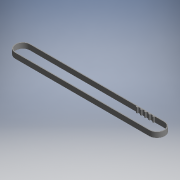
# Autodesk Inventor part: TBN154XL025_info-1-11-11
Saved by Autodesk Inventor 2017.3 (Build 213256000, 256)
## iProperties
Part Number: TBN154XL025_info-1-11-11
Material: Generic
Catalog Web Link: www.cadenas.de
Description: TBN__XL, TUN__XL-Timing Belts XL (Pitch : 5.08mm)
Vendor: MISUMI
Document SubType Name: Modeling
Designer: partserver
Manufacturer: MISUMI
Mass: 2.59371 g
Surface Area: 58.8219 cm^2
Volume: 2.59371 cm^3
Density: 1 g/cm^3
Appearance: PSOLRGB-175-175-175
Category: PARTsolutions
Company: MISUMI
Title: TBN154XL025
Author: Cadenas PARTsolutions
Comments: Timing Belts XL (Pitch : 5.08mm)
PSOL_IDENT_0: {$CADENAS_DATA\23d-libs\misumi\metric\48_timing_belts\tbn_xl.prj},213 {VTYP=3D},{NB=TBN154XL025_info
PSOL_IDENT_1: -1-11-11},{LINA=TBN154XL025},{NN=TBN__XL, TUN__XL},{DATE=08.06.2021 08:28:57},{GEOMDATE=07.05.2015 0
PSOL_IDENT_2: 7:10:15},{VERSION=},{LINEID=10},{WBVAR=TS,NT,RSSP,NT1,NT2},{WBNUMERIC=NT,NT1,NT2}  {NB=TBN154XL025_i
PSOL_IDENT_3: nfo-1-11-11},{LINA=TBN154XL025},{KT=DUMMY},{PN=TBN154XL025},{TS=TBN},{MATTC=Nylon Cloth},{MATTR=Neop
PSOL_IDENT_4: rene Rubber},{OT=-30~90},{MATCW=Glass Fiber Cord},{BNO=154XL},{BNW=6.4},{NT=77},{NTALG=30,34,35,38,3
PSOL_IDENT_5: 9,40,42,44,45,46,47,48,49,50,51,52,54,55,56,57,58,59,60,61,62,63,64,65,67,68,69,70,71,72,73,74,75,76
PSOL_IDENT_6: ,77,78,79,80,81,82,83,84,85,86,87,88,89,90,91,92,94,95,97,98,99,100,101,103,105,106,110,114,115,117,
PSOL_IDENT_7: 120,125,130,135,138,140,141,145,150,155,157,160,165,170,174,176,180,185,188,192,194,195,198,212,230,
PSOL_IDENT_8: 245,282,296,315,414,430},{BC=391.16},{PITCH=5.08},{ANGLE=50},{LRR=2.57},{HH=1.27},{H=2.27},{RRR=0.38
PSOL_IDENT_9: },{RAA=0.38},{BNWALG=025},{NTPN=154},{RSSP=1},{RSSP1= '1', '900 or Less', '2', 'Over 900, 1200 or Le
PSOL_IDENT_10: ss', '3'  , 'Over 1200, 1800 or Less', '4', 'Over 1800, 3600 or Less', '5'  , 'Over 3600, 4800 or Le
PSOL_IDENT_11: ss' },{NT1=11},{NT1A=11,12,14,15,16,18,19,20,21,22,24,25,26,28,30},{NT1A0=11,12,14,15,16,18,19,20,21
PSOL_IDENT_12: ,22,24,25,26,28,30},{NT1A1=0},{NT2=11},{NT2A=11,12,14,15,16,18,19,20,21,22,24,25,26,28,30,32,34,36,3
PSOL_IDENT_13: 8,40,42,44,46,48,50,60,72},{DRIVEP=17.78716},{DRIVENP=17.78716},{DRP=17.28},{DRNP=17.28},{BB=670.560
PSOL_IDENT_14: 00},{C=167.64},{NOTE=-},{ASSCFGC=NT2,C},{ASSCFGCNOTE=-},{FS=24.00},{FL=24.00},{CA=180.01},{ZM=-},{ZM
PSOL_IDENT_15: 1=5.5},{NT1SCR=11,12,14,15,16,18,19,20,21,22,24,25,26,28,30},{NT2SCR=11,12,14,15,16,18,19,20,21,22,2
PSOL_IDENT_16: 4,25,26,28,30,32,34,36,38,40,42,44,46,48,50,60,72}
NB: TBN154XL025_info-1-11-11
NN: TBN__XL, TUN__XL
NT: 77
NBSYN: $PN._info-$RSSP.-$NT1.-$NT2.
LINA: TBN154XL025
CATALOG: Misumi
PN: TBN154XL025
TS: Rubber
MATTC: Nylon Cloth
MATTR: Neoprene Rubber
OT: -30~90
MATCW: Glass Fiber Cord
BNO: 154XL
BNW: 6.4
BC: 391.16
PITCH: 5.08
ANGLE: 50
LRR: 2.57
HH: 1.27
H: 2.27
RRR: 0.38
RAA: 0.38
RSSP: 900 or Less
NT1: 11
NT2: 11
C: 167.64
NOTE: -
SUPPLIER: MISUMI
ARTICLENO: TBN154XL025_info-1-11-11
BOMINFO: TBN154XL025
CREATOR: CADENAS GmbH
Autodesk Inventor part; units mm, degrees
ref_plane "YZ Plane" through (0, 0, 0) normal (1, 0, 0) x (0, 1, 0)
ref_plane "XZ Plane" through (0, 0, 0) normal (0, 1, 0) x (-1, 0, 0)
ref_plane "XY Plane" through (0, 0, 0) normal (0, 0, 1) x (1, 0, 0)
sketch "Sketch_1" plane through (0, 0, 0) normal (0, 0, 1) x (1, 0, 0)
  line L0 (10.16, 8.64) -> (11.1729, 8.64)
  arc A0 (11.5173, 8.4206) -> (11.1729, 8.64) centre (11.1729, 8.26) ccw
  line L1 (11.5173, 8.4206) -> (11.9049, 7.5894)
  arc A1 (11.9049, 7.5894) -> (12.2493, 7.37) centre (12.2493, 7.75) ccw
  line L2 (12.2493, 7.37) -> (13.1507, 7.37)
  arc A2 (13.1507, 7.37) -> (13.4951, 7.5894) centre (13.1507, 7.75) ccw
  line L3 (13.4951, 7.5894) -> (13.8827, 8.4206)
  arc A3 (14.2271, 8.64) -> (13.8827, 8.4206) centre (14.2271, 8.26) ccw
  line L4 (14.2271, 8.64) -> (16.2529, 8.64)
  arc A4 (16.5973, 8.4206) -> (16.2529, 8.64) centre (16.2529, 8.26) ccw
  line L5 (16.5973, 8.4206) -> (16.9849, 7.5894)
  arc A5 (16.9849, 7.5894) -> (17.3293, 7.37) centre (17.3293, 7.75) ccw
  line L6 (17.3293, 7.37) -> (18.2307, 7.37)
  arc A6 (18.2307, 7.37) -> (18.5751, 7.5894) centre (18.2307, 7.75) ccw
  line L7 (18.5751, 7.5894) -> (18.9627, 8.4206)
  arc A7 (19.3071, 8.64) -> (18.9627, 8.4206) centre (19.3071, 8.26) ccw
  line L8 (19.3071, 8.64) -> (21.3329, 8.64)
  arc A8 (21.6773, 8.4206) -> (21.3329, 8.64) centre (21.3329, 8.26) ccw
  line L9 (21.6773, 8.4206) -> (22.0649, 7.5894)
  arc A9 (22.0649, 7.5894) -> (22.4093, 7.37) centre (22.4093, 7.75) ccw
  line L10 (22.4093, 7.37) -> (23.3107, 7.37)
  arc A10 (23.3107, 7.37) -> (23.6551, 7.5894) centre (23.3107, 7.75) ccw
  line L11 (23.6551, 7.5894) -> (24.0427, 8.4206)
  arc A11 (24.3871, 8.64) -> (24.0427, 8.4206) centre (24.3871, 8.26) ccw
  line L12 (24.3871, 8.64) -> (26.4129, 8.64)
  arc A12 (26.7573, 8.4206) -> (26.4129, 8.64) centre (26.4129, 8.26) ccw
  line L13 (26.7573, 8.4206) -> (27.1449, 7.5894)
  arc A13 (27.1449, 7.5894) -> (27.4893, 7.37) centre (27.4893, 7.75) ccw
  line L14 (27.4893, 7.37) -> (28.3907, 7.37)
  arc A14 (28.3907, 7.37) -> (28.7351, 7.5894) centre (28.3907, 7.75) ccw
  line L15 (28.7351, 7.5894) -> (29.1227, 8.4206)
  arc A15 (29.4671, 8.64) -> (29.1227, 8.4206) centre (29.4671, 8.26) ccw
  line L16 (29.4671, 8.64) -> (31.4929, 8.64)
  arc A16 (31.8373, 8.4206) -> (31.4929, 8.64) centre (31.4929, 8.26) ccw
  line L17 (31.8373, 8.4206) -> (32.2249, 7.5894)
  arc A17 (32.2249, 7.5894) -> (32.5693, 7.37) centre (32.5693, 7.75) ccw
  line L18 (32.5693, 7.37) -> (33.4707, 7.37)
  arc A18 (33.4707, 7.37) -> (33.8151, 7.5894) centre (33.4707, 7.75) ccw
  line L19 (33.8151, 7.5894) -> (34.2027, 8.4206)
  arc A19 (34.5471, 8.64) -> (34.2027, 8.4206) centre (34.5471, 8.26) ccw
  line L20 (34.5471, 8.64) -> (35.56, 8.64)
  line L21 (35.56, 8.64) -> (35.56, 9.24)
  line L22 (35.56, 9.24) -> (10.16, 9.24)
  line L23 (10.16, 9.24) -> (10.16, 8.64)
  constraints: 48 end point, 40 point on circle, 20 centre point
extrude "Extrusion1" add sketch "Sketch_1" along normal mid plane 6.4
sketch "Sketch_2" plane through (0, 0, 0) normal (0, 0, 1) x (1, 0, 0)
  arc A0 (0, 9.64) -> (0, -9.64) centre (0, 0) ccw
  line L0 (0, -9.64) -> (167.64, -9.64)
  arc A1 (167.64, -9.64) -> (167.64, 9.64) centre (167.64, 0) ccw
  line L1 (167.64, 9.64) -> (0, 9.64)
  arc A2 (0, 8.64) -> (0, -8.64) centre (0, 0) ccw
  line L2 (0, -8.64) -> (167.64, -8.64)
  arc A3 (167.64, -8.64) -> (167.64, 8.64) centre (167.64, 0) ccw
  line L3 (167.64, 8.64) -> (0, 8.64)
  constraints: 8 end point, 8 point on circle, 4 centre point
extrude "Extrusion2" add sketch "Sketch_2" along normal mid plane 6.4
body "Solid1"
